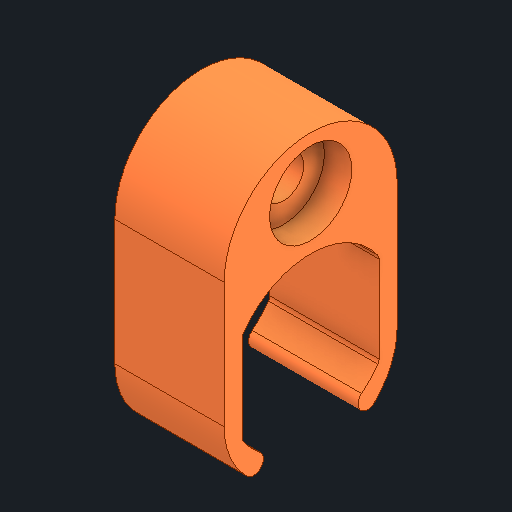
# Autodesk Inventor part: X Stage Motor Clamp V5
Saved by Autodesk Inventor 2023.4 (Build 274418000, 418)
## iProperties
Created: 2024-05-29
Part Number: X Stage Motor Clamp V5
Material: Generic
Document SubType Name: Modeling
Designer: xSibe
Density: 1 g/cm^3
Appearance: Plastic Orange
Author: xSibe
Autodesk Inventor part; units mm, degrees
ref_plane "YZ Plane" through (0, 0, 0) normal (1, 0, 0) x (0, 1, 0)
ref_plane "XZ Plane" through (0, 0, 0) normal (0, 1, 0) x (-1, 0, 0)
sketch "Sketch1" plane through (0, 0, 0) normal (1, 0, 0) x (0, 1, 0)
  line L0 (14.875, -0.7) -> (14.875, 0.8967) projected
  line L1 (27.025, -0.7) -> (14.875, -0.7) projected
  line L2 (27.025, -10.85) -> (27.025, -0.7) projected
  line L3 (15.75, -10.85) -> (27.025, -10.85) projected
  line L4 (34.625, -12.1) -> (15.75, -12.1) projected
  line L5 (34.625, -3.2) -> (34.625, -12.1) projected
  line L6 (15.7197, 0.55) -> (30.875, 0.55) projected
  arc A0 (17.7877, -0.775) -> (17.5002, -0.8659) centre (17.7877, -1.275) ccw projected
  arc A1 (17.5002, -0.8659) -> (17.5002, -10.6841) centre (20.95, -5.775) ccw projected
  arc A2 (17.5002, -10.6841) -> (17.7877, -10.775) centre (17.7877, -10.275) ccw projected
  line L7 (17.7877, -10.775) -> (24.1123, -10.775) projected
  arc A3 (24.1123, -10.775) -> (24.3998, -10.6841) centre (24.1123, -10.275) ccw projected
  arc A4 (24.3998, -10.6841) -> (24.3998, -0.8659) centre (20.95, -5.775) ccw projected
  arc A5 (24.3998, -0.8659) -> (24.1123, -0.775) centre (24.1123, -1.275) ccw projected
  line L8 (24.1123, -0.775) -> (17.7877, -0.775) projected
  line L9 (26.95, -5.775) -> (26.95, -9.775) projected
  arc A6 (24.3998, -10.6841) -> (26.95, -5.775) centre (20.95, -5.775) ccw projected
  arc A7 (24.1123, -10.775) -> (24.3998, -10.6841) centre (24.1123, -10.275) ccw projected
  line L10 (25.95, -10.775) -> (24.1123, -10.775) projected
  arc A8 (25.95, -10.775) -> (26.95, -9.775) centre (25.95, -9.775) ccw projected
  line L11 (24.1123, -0.775) -> (25.95, -0.775) projected
  arc A9 (24.3998, -0.8659) -> (24.1123, -0.775) centre (24.1123, -1.275) ccw projected
  arc A10 (26.95, -5.775) -> (24.3998, -0.8659) centre (20.95, -5.775) ccw projected
  line L12 (26.95, -1.775) -> (26.95, -5.775) projected
  arc A11 (26.95, -1.775) -> (25.95, -0.775) centre (25.95, -1.775) ccw projected
  line L13 (14.95, -5.775) -> (14.95, -1.775) projected
  arc A12 (17.5002, -0.8659) -> (14.95, -5.775) centre (20.95, -5.775) ccw projected
  arc A13 (17.7877, -0.775) -> (17.5002, -0.8659) centre (17.7877, -1.275) ccw projected
  line L14 (15.95, -0.775) -> (17.7877, -0.775) projected
  arc A14 (15.95, -0.775) -> (14.95, -1.775) centre (15.95, -1.775) ccw projected
  line L15 (17.7877, -10.775) -> (15.95, -10.775) projected
  arc A15 (17.5002, -10.6841) -> (17.7877, -10.775) centre (17.7877, -10.275) ccw projected
  arc A16 (14.95, -5.775) -> (17.5002, -10.6841) centre (20.95, -5.775) ccw projected
  line L16 (14.95, -9.775) -> (14.95, -5.775) projected
  arc A17 (14.95, -9.775) -> (15.95, -10.775) centre (15.95, -9.775) ccw projected
  line L17 (26.95, -10.85) -> (14.95, -10.85)
  line L18 (14.95, -10.85) -> (14.95, -12.1)
  line L19 (14.95, -12.1) -> (26.95, -12.1)
  line L20 (26.95, -12.1) -> (26.95, -10.85)
  line L21 (20.95, -5.775) -> (14.95, -5.775)
  arc A18 (15.2429, -10.4821) -> (19.1488, -12.1) centre (19.1488, -6.5762) ccw
  arc A19 (15.8269, -8.8981) -> (14.95, -9.775) centre (15.8269, -9.775) ccw
  line L22 (14.95, -9.775) -> (15.8269, -8.8981) construction
  line L23 (14.95, -9.775) -> (16.1901, -9.775) construction
  line L24 (26.95, -0.7) -> (14.95, -0.7)
  line L25 (14.95, -0.7) -> (14.95, 0.55)
  line L26 (14.95, 0.55) -> (26.95, 0.55)
  line L27 (26.95, 0.55) -> (26.95, -0.7)
  arc A20 (19.1488, 0.55) -> (15.2429, -1.0679) centre (19.1488, -4.9738) ccw
  arc A21 (14.95, -1.775) -> (15.8269, -2.6519) centre (15.8269, -1.775) ccw
  line L28 (26.95, -12.1) -> (26.95, 0.55)
  line L29 (26.95, 0.55) -> (34.625, 0.55)
  line L30 (34.625, 0.55) -> (34.625, -12.1)
  line L31 (34.625, -12.1) -> (26.95, -12.1)
  line L32 (26.95, -5.775) -> (34.625, -5.775)
  circle A22 centre (30.7875, -5.775) radius 1.5
  circle A23 centre (30.7875, -5.775) radius 3
  arc A24 (28.3, -12.1) -> (34.625, -5.775) centre (28.3, -5.775) ccw
  arc A25 (34.625, -5.775) -> (28.3, 0.55) centre (28.3, -5.775) ccw
  line L33 (15.75, -12.1) -> (15.75, -10.85) projected
  arc A26 (34.625, -3.2) -> (30.875, 0.55) centre (30.875, -3.2) ccw projected
  arc A27 (14.8505, 1.3251) -> (15.7197, 0.55) centre (15.7197, 1.425) ccw projected
  arc A28 (14.875, 0.8967) -> (14.8505, 1.3251) centre (11.125, 0.8967) ccw projected
  circle A29 centre (30.7875, -5.775) radius 1.4375 projected
  point P0 (0, 0)
  point P1 (15.8269, -8.8981)
  point P2 (19.1488, -12.1)
  point P3 (28.3, -12.1)
  point P4 (28.3, 0.55)
  point P5 (19.1488, 0.55)
  point P6 (15.2429, -1.0679)
  point P7 (15.8269, -2.6519)
  point P8 (15.75, -10.9306)
  point P9 (27.025, -5.775)
  point P10 (15.6492, -0.7)
  dimension "d0" = 1.25
  dimension "d1" = 45
  dimension "d2" = 3
  dimension "d3" = 6
  constraints: 32 end point, 14 point on circle, 9 symmetric about line, 8 centre point, 7 tangent, 4 parallel, 4 perpendicular, 4 point on line, 3 collinear, 2 midpoint, 1 coincident, 1 equal length, 1 horizontal, 6 other
  measures "d0" distance of L18.end L17.end
  measures "d1" angle of L23 L22
  measures "d2" diameter of A22
  measures "d3" diameter of A23
ref_plane "Work Plane1" through (124.425, 27.025, -10.85) normal (1, 0, 0) x (0, 1, 0)
extrude "Extrusion1" add sketch "Sketch1" along normal blind 6 from surface at 124.425 contours A20 L6 L27 L1 | L1 L28 A11 L11 L8 L14 A14 A20 | L27 L6 A25 L32 A23 L2 L1 | L1 L2 L32 L12 L28 | A14 L14 A0 A1 A21 | L12 A4 A5 L11 A11 | L32 A23 A24 L4 L20 L3 L2 | L2 L3 L28 L9 L32 | L9 A8 L10 A3 A4 | A23 L32 A22 | L32 A22 A23 | L28 L3 L17 A18 A17 L15 L7 L10 A8 | A1 A2 L15 A17 A19 | L20 L4 A18 L33 L3 | L33 A18 L17
fillet "Fillet1" radius 0.7 2 edges at (127.425, 15.8269, -2.6519) (127.425, 15.8269, -8.8981)
sketch "Sketch2" plane through (130.425, 19.1488, -12.1) normal (1, 0, 0) x (0, 0, -1)
  arc A0 (-2.6078, -2.9087) -> (-1.8221, -4.0632) centre (-2.1741, -3.4581) ccw projected
  line L0 (0, 9.1512) -> (0, 0) projected
  line L1 (-12.65, 0) -> (-12.65, 9.1512) projected
  arc A1 (-11.0321, -3.9059) -> (-10.8279, -4.0632) centre (-10.325, -3.1988) ccw projected
  arc A2 (-11.2341, -1.6486) -> (-10.0422, -2.9087) centre (-6.325, 1.8012) ccw projected
  arc A3 (-11.325, -1.3611) -> (-11.2341, -1.6486) centre (-10.825, -1.3611) ccw projected
  arc A4 (-2.6078, -2.9087) -> (-1.4159, -1.6486) centre (-6.325, 1.8012) ccw projected
  circle A5 centre (-6.325, 11.6387) radius 1.5 projected
  circle A6 centre (-6.325, 11.6387) radius 3
  arc A7 (-1.8221, -4.0632) -> (-1.6179, -3.9059) centre (-2.325, -3.1988) ccw projected
  arc A8 (-1.6179, -3.9059) -> (0, 0) centre (-5.5238, 0) ccw projected
  arc A9 (0, 9.1512) -> (-12.65, 9.1512) centre (-6.325, 9.1512) ccw projected
  arc A10 (-12.65, 0) -> (-11.0321, -3.9059) centre (-7.1262, 0) ccw projected
  arc A11 (-10.8279, -4.0632) -> (-10.0422, -2.9087) centre (-10.4759, -3.4581) ccw projected
  line L2 (-11.325, 4.9634) -> (-11.325, -1.3611) projected
  arc A12 (-11.2341, 5.2509) -> (-11.325, 4.9634) centre (-10.825, 4.9634) ccw projected
  arc A13 (-1.4159, 5.2509) -> (-11.2341, 5.2509) centre (-6.325, 1.8012) ccw projected
  arc A14 (-1.325, 4.9634) -> (-1.4159, 5.2509) centre (-1.825, 4.9634) ccw projected
  line L3 (-1.325, -1.3611) -> (-1.325, 4.9634) projected
  arc A15 (-1.4159, -1.6486) -> (-1.325, -1.3611) centre (-1.825, -1.3611) ccw projected
  point P0 (-12.1, -19.1488)
  dimension "d7" = 6
  constraints: 1 centre point, 1 coincident
  measures "d7" diameter of A6
extrude "Extrusion2" add sketch "Sketch2" along normal blind 2 contours A4 A15 L3 A14 A13 A12 L2 A3 A2 A11 A1 A10 L1 A9 L0 A8 A7 A0
body "Solid1"
